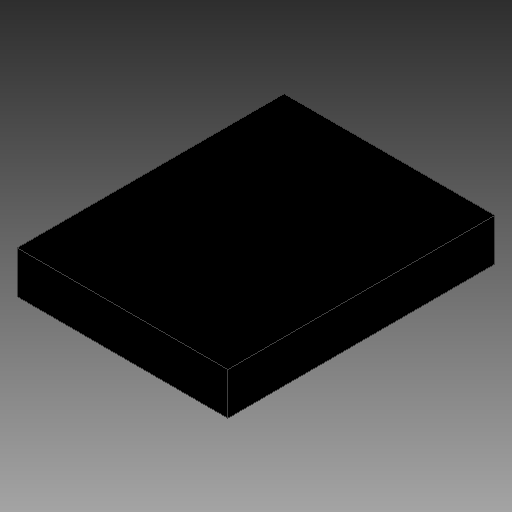
# Autodesk Inventor part: screen
Saved by Autodesk Inventor 2017 (Build 210142000, 142)
## iProperties
Created: 2019-03-27
Part Number: screen
Material: Generic
Document SubType Name: Modeling
Designer: Mitch
Density: 1 g/cm^3
Appearance: Anodized - Black
Mass: 1751.16 g
Surface Area: 1250.01 cm^2
Volume: 1751.16 cm^3
Author: Mitch
Autodesk Inventor part; units mm, degrees
ref_plane "YZ Plane" through (0, 0, 0) normal (1, 0, 0) x (0, 1, 0)
ref_plane "XZ Plane" through (0, 0, 0) normal (0, 1, 0) x (-1, 0, 0)
ref_plane "XY Plane" through (0, 0, 0) normal (0, 0, 1) x (1, 0, 0)
sketch "Sketch1" plane through (0, 0, 0) normal (0, 1, 0) x (-1, 0, 0)
  line L0 (0, 0) -> (190.5, 0)
  line L1 (190.5, 0) -> (190.5, -241.3)
  line L2 (190.5, -241.3) -> (0, -241.3)
  line L3 (0, -241.3) -> (0, 0)
  dimension "d0" = 190.5
  dimension "d1" = 241.3
  constraints: 8 end point, 2 parallel, 1 horizontal, 1 perpendicular
  measures "d0" distance of L1.end L2.end
  measures "d1" distance of L0.end L1.end
extrude "Extrusion1" add sketch "Sketch1" along normal blind 38.1
sketch "Sketch2" plane through (0, 0, 0) normal (0, -1, 0) x (1, 0, 0)
  circle A0 centre (-134.9375, -157.1625) radius 2.54
  line L0 (-190.5, 0) -> (-190.5, -241.3) projected
  line L1 (0, -241.3) -> (-190.5, -241.3) projected
  circle A1 centre (-60.325, -157.1625) radius 2.54
  circle A2 centre (-134.9375, -82.55) radius 2.54
  circle A3 centre (-60.325, -82.55) radius 2.54
  point P0 (0, 0)
  dimension "d4" = 5.08
  dimension "d5" = 55.5625
  dimension "d6" = 84.1375
  dimension "d7" = 5.08
  dimension "d8" = 5.08
  dimension "d9" = 74.6125
  dimension "d10" = 74.6125
  dimension "d11" = 5.08
  dimension "d12" = 74.6125
  dimension "d13" = 74.6125
  constraints: 4 centre point
  measures "d4" diameter of A0
  measures "d5" distance from line of A0.centre L0
  measures "d6" distance from line of L1 A0.centre
  measures "d7" diameter of A1
  measures "d8" diameter of A2
  measures "d9" distance of A2.centre A0.centre
  measures "d10" distance of A1.centre A0.centre
  measures "d11" diameter of A3
  measures "d12" distance of A3.centre A1.centre
  measures "d13" distance of A3.centre A2.centre
extrude "Extrusion2" cut sketch "Sketch2" against normal blind 2.54
body "Solid1"
